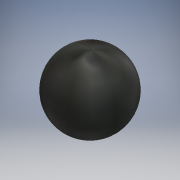
# Autodesk Inventor part: 12mmBallBearing
Saved by Autodesk Inventor 2018 (Build 220112000, 112)
## iProperties
Created: 2018-05-08
Part Number: 12mmBallBearing
Material: Steel
Document SubType Name: Modeling
Designer: P136265
Density: 7.85 g/cm^3
Appearance: Plate
Author: P136265
Autodesk Inventor part; units mm, degrees
ref_plane "YZ Plane" through (0, 0, 0) normal (1, 0, 0) x (0, 1, 0)
ref_plane "XZ Plane" through (0, 0, 0) normal (0, 1, 0) x (-1, 0, 0)
ref_plane "XY Plane" through (0, 0, 0) normal (0, 0, 1) x (1, 0, 0)
sketch "Sketch1" plane through (0, 0, 0) normal (0, 1, 0) x (-1, 0, 0)
  arc A0 (0, -1.394) -> (0, 1.394) centre (0, 0) ccw
  line L0 (0, 1.394) -> (0, -1.394)
  dimension "d0" = 2.788
  dimension "d1" = 0
  constraints: 2 end point, 2 point on circle, 1 centre point, 1 coincident, 1 vertical
  measures "d0" diameter of A0
  measures "d1" distance from line of point (0, 0) L0
revolve "Revolution1" add sketch "Sketch1" angle 360 about axis through (0, 0, 1.394) along (0, 0, -1)
body "Solid1"
